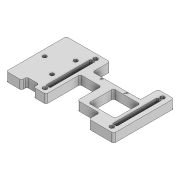
# Autodesk Inventor part: Bottom PMMA
Saved by Autodesk Inventor 2020 (Build 240168000, 168)
## iProperties
Created: 2021-07-01
Part Number: Bottom PMMA
Material: Generic
Document SubType Name: Modeling
Designer: ferrerx
Density: 1 g/cm^3
Appearance: Default
Author: ferrerx
Autodesk Inventor part; units mm, degrees
ref_plane "YZ Plane" through (0, 0, 0) normal (1, 0, 0) x (0, 1, 0)
ref_plane "XZ Plane" through (0, 0, 0) normal (0, 1, 0) x (-1, 0, 0)
ref_plane "XY Plane" through (0, 0, 0) normal (0, 0, 1) x (1, 0, 0)
sketch "Sketch1" plane through (0, 0, 0) normal (0, 1, 0) x (-1, 0, 0)
  line L0 (-2.27, 0) -> (120.44, 0)
  line L1 (120.44, 0) -> (120.44, -68.57)
  line L2 (120.44, -68.57) -> (-2.27, -68.57)
  line L3 (-2.27, -68.57) -> (-2.27, 0)
  line L4 (120.44, -66.57) -> (120.44, -2)
  line L5 (0, -68.57) -> (118.44, -68.57)
  line L6 (-2.27, -2.27) -> (-2.27, -66.3)
  circle A0 centre (81.55, -63.09) radius 1.5
  circle A1 centre (81.55, -63.09) radius 1.5
  line L7 (70.44, -68.57) -> (15.73, -68.57)
  line L8 (15.73, -68.57) -> (15.73, -48.57)
  line L9 (15.73, -48.57) -> (70.44, -48.57)
  line L10 (70.44, -48.57) -> (70.44, -68.57)
  line L11 (75, -39) -> (51, -39)
  line L12 (51, -39) -> (51, 0)
  line L13 (51, 0) -> (75, 0)
  line L14 (75, 0) -> (75, -39)
  line L15 (51, -12) -> (26, -12)
  line L16 (26, -12) -> (26, 0)
  line L17 (26, 0) -> (51, 0)
  line L18 (51, 0) -> (51, -12)
  line L19 (11.73, -15.57) -> (42, -15.57)
  line L20 (84, -60) -> (79, -60)
  line L21 (79, -60) -> (79, -8.7337)
  line L22 (79, -8.7337) -> (84, -8.7337)
  line L23 (84, -8.7337) -> (84, -60)
  line L24 (8, -60) -> (3, -60)
  line L25 (3, -60) -> (3, -8.7337)
  line L26 (3, -8.7337) -> (8, -8.7337)
  line L27 (8, -8.7337) -> (8, -60)
  circle A2 centre (5.25, -63.09) radius 1.5
  circle A3 centre (5.35, -5.47) radius 1.5
  circle A4 centre (81.55, -5.47) radius 1.5
  circle A5 centre (81.55, -5.47) radius 1.5
  circle A6 centre (5.35, -5.47) radius 1.5
  circle A7 centre (5.25, -63.09) radius 1.5
  line L28 (42, -15.57) -> (42, -44)
  line L29 (42, -44) -> (11.73, -44)
  line L30 (11.73, -44) -> (11.73, -15.57)
  dimension "d20" = 3
  dimension "d21" = 18
  dimension "d22" = 50
  dimension "d23" = 12
  dimension "d24" = 30.27
  dimension "d25" = 24
  dimension "d26" = 39
  dimension "d27" = 3
  dimension "d28" = 3
  dimension "d29" = 3
  dimension "d30" = 68.57
  dimension "d31" = 20
  dimension "d32" = 28.43
  dimension "d33" = 30.27
  constraints: 62 end point, 12 parallel, 8 centre point, 8 perpendicular, 6 horizontal, 4 collinear, 4 concentric, 4 point on line, 1 vertical
  measures "d20" diameter of A0
  measures "d21" distance between parallel lines of L3 L8
  measures "d22" distance between parallel lines of L1 L10
  measures "d23" distance of L15.end L16.end
  measures "d24" distance of L30.end L19.end
  measures "d25" distance of L11.start L12.start
  measures "d26" distance of L13.end L11.start
  measures "d27" diameter of A2
  measures "d28" diameter of A3
  measures "d29" diameter of A4
  measures "d30" distance of L0.end L1.end
  measures "d31" distance of L7.end L9.start
  measures "d32" distance of L29.end L30.end
  measures "d33" distance of L29.start L29.end
extrude "Extrusion1" add sketch "Sketch1" along normal blind 10 contours L0 L16 L15 L12 L11 L14 L1 L2 L10 L9 L8 L3
fillet "Fillet4" radius 2 4 edges at (-120.44, 5, -68.57) (-120.44, 5, 0) (2.27, 5, -68.57) (2.27, 5, 0)
fillet "Fillet5" radius 2 14 edges at (-70.44, 5, -68.57) (-70.44, 5, -48.57) (-15.73, 5, -68.57) (-15.73, 5, -48.57) (-11.73, 5, -44) (-11.73, 5, -15.57) (-42, 5, -15.57) (-42, 5, -44) (-26, 5, -12) (-51, 5, -12) (-26, 5, 0) (-51, 5, -39) (-75, 5, -39) (-75, 5, 0)
fillet "Fillet6" radius 1 8 edges at (-8, 5, -8.7337) (-3, 5, -8.7337) (-3, 5, -60) (-8, 5, -60) (-79, 5, -8.7337) (-84, 5, -8.7337) (-84, 5, -60) (-79, 5, -60)
sketch "Sketch2" plane through (0, 10, 0) normal (0, 1, 0) x (1, 0, 0)
  line L0 (-31.8779, 47.8881) -> (-29.0182, 47.8881) construction
  line L1 (-29.0182, 47.8881) -> (-29.0182, 44.8381) construction
  line L2 (-29.0182, 44.8381) -> (-31.8779, 44.8381) construction
  line L3 (-31.8779, 44.8381) -> (-31.8779, 47.8881) construction
  line L4 (-60.0668, 48.1942) -> (-57.2071, 48.1942) construction
  line L5 (-57.2071, 48.1942) -> (-57.2071, 45.1442) construction
  line L6 (-57.2071, 45.1442) -> (-60.0668, 45.1442) construction
  line L7 (-60.0668, 45.1442) -> (-60.0668, 48.1942) construction
  line L8 (-28.8304, 47.5273) -> (-30.2491, 47.5273)
  line L9 (-30.2491, 47.5273) -> (-30.5432, 46.6671)
  line L10 (-30.5432, 46.6671) -> (-29.1838, 46.6671)
  line L11 (-29.1838, 46.6671) -> (-29.3049, 46.3063)
  line L12 (-29.3049, 46.3063) -> (-30.6643, 46.3063)
  line L13 (-30.6643, 46.3063) -> (-31.1636, 44.8381)
  line L14 (-31.1636, 44.8381) -> (-31.5689, 44.8381)
  line L15 (-31.5689, 44.8381) -> (-30.5333, 47.8881)
  line L16 (-30.5333, 47.8881) -> (-28.7093, 47.8881)
  line L17 (-28.7093, 47.8881) -> (-28.8304, 47.5273)
  line L18 (-57.212, 47.8135) -> (-58.8532, 45.5248)
  line L19 (-58.8532, 45.5248) -> (-59.1992, 45.5248)
  line L20 (-59.1992, 45.5248) -> (-59.2759, 47.8135)
  line L21 (-59.2759, 47.8135) -> (-58.8606, 47.8135)
  line L22 (-58.8606, 47.8135) -> (-58.8334, 46.0513)
  line L23 (-58.8334, 46.0513) -> (-57.6149, 47.8135)
  line L24 (-57.6149, 47.8135) -> (-57.212, 47.8135)
  point P0 (0, 0)
  constraints: 4 other
emboss "Emboss1" sketch "Sketch2" operation cut depth 1 direction (0, -1, 0)
sketch "Sketch3" plane through (0, 10, 0) normal (0, 1, 0) x (1, 0, 0)
  line L0 (-118.44, 0) -> (-77, 0) projected
  line L1 (-88.94, 0) -> (-102.94, 0)
  line L2 (-102.94, 0) -> (-102.94, 6)
  line L3 (-102.94, 6) -> (-88.94, 6)
  line L4 (-88.94, 6) -> (-88.94, 0)
  line L5 (-120.44, 66.57) -> (-120.44, 2) projected
  point P0 (0, 0)
  point P1 (-102.94, 0)
  dimension "d39" = 17.5
  dimension "d40" = 6
  dimension "d43" = 14
  constraints: 8 end point, 2 parallel, 1 horizontal, 1 perpendicular, 1 point on line
  measures "d39" distance between parallel lines of L5 L2
  measures "d40" distance of L3.end L1.start
  measures "d43" distance of L2.end L3.end
extrude "Extrusion2" cut sketch "Sketch3" against normal blind 10
fillet "Fillet7" radius 2 4 edges at (-88.94, 5, 0) (-88.94, 5, -6) (-102.94, 5, -6) (-102.94, 5, 0)
sketch "Sketch4" plane through (0, 10, 0) normal (0, 1, 0) x (1, 0, 0)
  circle A0 centre (-91.14, 23.07) radius 1.25
  circle A1 centre (-91.14, 50.07) radius 1.25
  circle A2 centre (-113.14, 36.57) radius 1.25
  line L0 (-72.44, 68.57) -> (-118.44, 68.57) projected
  line L1 (-120.44, 66.57) -> (-120.44, 2) projected
  point P0 (0, 0)
  dimension "d45" = 27
  dimension "d46" = 22
  dimension "d47" = 2.5
  dimension "d48" = 2.5
  dimension "d49" = 2.5
  dimension "d50" = 22
  dimension "d51" = 13.5
  dimension "d52" = 18.5
  dimension "d53" = 7.3
  constraints: 3 centre point
  measures "d45" distance of A0.centre A1.centre
  measures "d46" horizontal distance of A2.centre A1.centre
  measures "d47" diameter of A2
  measures "d48" diameter of A0
  measures "d49" diameter of A1
  measures "d50" horizontal distance of A2.centre A0.centre
  measures "d51" vertical distance of A1.centre A2.centre
  measures "d52" distance from line of L0 A1.centre
  measures "d53" distance from line of L1 A2.centre
extrude "Extrusion3" cut sketch "Sketch4" against normal blind 10
sketch "Sketch5" plane through (0, 10, 0) normal (0, 1, 0) x (1, 0, 0)
  circle A0 centre (-113.14, 36.57) radius 1.25 projected
  line L0 (-115.4494, 36.57) -> (-114.2947, 38.57)
  line L1 (-114.2947, 38.57) -> (-111.9853, 38.57)
  line L2 (-111.9853, 38.57) -> (-110.8306, 36.57)
  line L3 (-110.8306, 36.57) -> (-111.9853, 34.57)
  line L4 (-111.9853, 34.57) -> (-114.2947, 34.57)
  line L5 (-114.2947, 34.57) -> (-115.4494, 36.57)
  circle A1 centre (-91.14, 23.07) radius 1.25 projected
  line L6 (-93.4494, 23.07) -> (-92.2947, 25.07)
  line L7 (-92.2947, 25.07) -> (-89.9853, 25.07)
  line L8 (-89.9853, 25.07) -> (-88.8306, 23.07)
  line L9 (-88.8306, 23.07) -> (-89.9853, 21.07)
  line L10 (-89.9853, 21.07) -> (-92.2947, 21.07)
  line L11 (-92.2947, 21.07) -> (-93.4494, 23.07)
  circle A2 centre (-91.14, 50.07) radius 1.25 projected
  line L12 (-93.4494, 50.07) -> (-92.2947, 52.07)
  line L13 (-92.2947, 52.07) -> (-89.9853, 52.07)
  line L14 (-89.9853, 52.07) -> (-88.8306, 50.07)
  line L15 (-88.8306, 50.07) -> (-89.9853, 48.07)
  line L16 (-89.9853, 48.07) -> (-92.2947, 48.07)
  line L17 (-92.2947, 48.07) -> (-93.4494, 50.07)
  point P0 (0, 0)
  dimension "d56" = 4
  dimension "d57" = 4
  dimension "d58" = 4
  constraints: 36 end point, 3 coincident, 39 other
  measures "d56" distance between parallel lines of L10 L7
  measures "d57" distance between parallel lines of L4 L1
  measures "d58" distance between parallel lines of L16 L13
extrude "Extrusion4" cut sketch "Sketch5" against normal blind 10
sketch "Sketch6" plane through (0, 10, 0) normal (0, 1, 0) x (1, 0, 0)
  circle A0 centre (-5.35, 5.47) radius 1.5 projected
  line L0 (-7.9481, 5.47) -> (-6.649, 7.72)
  line L1 (-6.649, 7.72) -> (-4.051, 7.72)
  line L2 (-4.051, 7.72) -> (-2.7519, 5.47)
  line L3 (-2.7519, 5.47) -> (-4.051, 3.22)
  line L4 (-4.051, 3.22) -> (-6.649, 3.22)
  line L5 (-6.649, 3.22) -> (-7.9481, 5.47)
  circle A1 centre (-5.25, 63.09) radius 1.5 projected
  line L6 (-7.8481, 63.09) -> (-6.549, 65.34)
  line L7 (-6.549, 65.34) -> (-3.951, 65.34)
  line L8 (-3.951, 65.34) -> (-2.6519, 63.09)
  line L9 (-2.6519, 63.09) -> (-3.951, 60.84)
  line L10 (-3.951, 60.84) -> (-6.549, 60.84)
  line L11 (-6.549, 60.84) -> (-7.8481, 63.09)
  circle A2 centre (-81.55, 63.09) radius 1.5 projected
  line L12 (-84.1481, 63.09) -> (-82.849, 65.34)
  line L13 (-82.849, 65.34) -> (-80.251, 65.34)
  line L14 (-80.251, 65.34) -> (-78.9519, 63.09)
  line L15 (-78.9519, 63.09) -> (-80.251, 60.84)
  line L16 (-80.251, 60.84) -> (-82.849, 60.84)
  line L17 (-82.849, 60.84) -> (-84.1481, 63.09)
  circle A3 centre (-81.55, 5.47) radius 1.5 projected
  line L18 (-82.849, 7.72) -> (-80.251, 7.72)
  line L19 (-80.251, 7.72) -> (-78.9519, 5.47)
  line L20 (-78.9519, 5.47) -> (-80.251, 3.22)
  line L21 (-80.251, 3.22) -> (-82.849, 3.22)
  line L22 (-82.849, 3.22) -> (-84.1481, 5.47)
  line L23 (-84.1481, 5.47) -> (-82.849, 7.72)
  line L24 (-86.94, 0) -> (-77, 0) projected
  point P0 (0, 0)
  dimension "d61" = 4.5
  dimension "d62" = 4.5
  dimension "d63" = 4.5
  dimension "d64" = 4.5
  constraints: 48 end point, 4 coincident, 1 parallel, 52 other
  measures "d61" distance between parallel lines of L18 L21
  measures "d62" distance between parallel lines of L4 L1
  measures "d63" distance between parallel lines of L7 L10
  measures "d64" distance between parallel lines of L16 L13
extrude "Extrusion5" cut sketch "Sketch6" against normal blind 10
body "Solid1"
